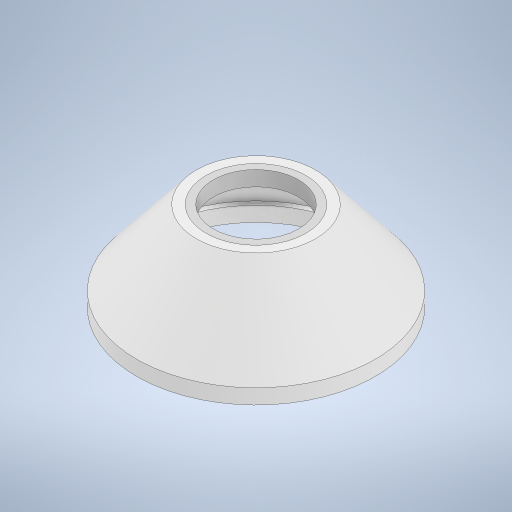
# Autodesk Inventor part: Parte baja R2D2
Saved by Autodesk Inventor 2023 (Build 270158000, 158)
## iProperties
Created: 2022-10-09
Part Number: Parte baja R2D2
Material: Generic
Document SubType Name: Modeling
Designer: User
Density: 1 g/cm^3
Appearance: Default
Author: User
## iProperties of the stored document Parte baja R2D2_3DPrint.ipt
Created: 2022-10-19
Part Number: Parte baja R2D2_3DPrint
Material: Generic
Document SubType Name: Modeling
Designer: User
Density: 1 g/cm^3
Appearance: Default
Author: User
Autodesk Inventor part; units mm, degrees
ref_plane "YZ Plane" through (0, 0, 0) normal (1, 0, 0) x (0, 1, 0)
ref_plane "XZ Plane" through (0, 0, 0) normal (0, 1, 0) x (-1, 0, 0)
ref_plane "XY Plane" through (0, 0, 0) normal (0, 0, 1) x (1, 0, 0)
sketch "Sketch1" plane through (0, 0, 0) normal (0, 1, 0) x (-1, 0, 0)
  circle A0 centre (0, 0) radius 80
  circle A1 centre (0, 0) radius 70
  dimension "d0" = 160
  dimension "d1" = 10
  constraints: 2 centre point, 2 coincident
  measures "d0" diameter of A0
  measures "d1" radial gap between concentric circles of A0 A1
extrude "Extrusion1" add sketch "Sketch1" along normal blind 10
ref_plane "Work Plane1" through (0, 60, 0) normal (0, 1, 0) x (1, 0, 0)
sketch "Sketch2" plane through (0, 60, 0) normal (0, 1, 0) x (1, 0, 0)
  circle A0 centre (0, 0) radius 45
  circle A1 centre (0, 0) radius 70 projected
  circle A2 centre (0, 0) radius 40
  dimension "d5" = 25
  dimension "d6" = 5
  constraints: 2 centre point, 2 coincident
  measures "d5" radial gap between concentric circles of A0 A1
  measures "d6" radial gap between concentric circles of A0 A2
loft "Loft1" add profiles "Sketch2" section 1 edges at (80, 10, 0) contours A2
shell "Shell1" thickness 5 removed faces 2 at (11.6583, 60, -8.2987) at (-10.1521, 10, 16.6986)
sketch "Sketch4" plane through (0, 60, 0) normal (0, 1, 0) x (1, 0, 0)
  circle A0 centre (0, 0) radius 28.5969
  circle A1 centre (0, 0) radius 33.5969 projected
  dimension "d18" = 5
  constraints: 1 centre point, 1 coincident
  measures "d18" radial gap between concentric circles of A1 A0
extrude "Extrusion4" add sketch "Sketch4" against normal blind 10
body "Solid1"
